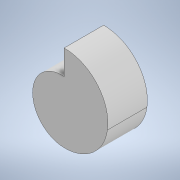
# Autodesk Inventor part: Snail Cam
Saved by Autodesk Inventor 2021 (Build 250183000, 183)
## iProperties
Created: 2021-03-30
Part Number: Snail Cam
Material: Generic
Document SubType Name: Modeling
Designer: Nabeel Azafer
Density: 1 g/cm^3
Appearance: Default
Author: Nabeel Azafer
Autodesk Inventor part; units mm, degrees
ref_plane "YZ Plane" through (0, 0, 0) normal (1, 0, 0) x (0, 1, 0)
ref_plane "XZ Plane" through (0, 0, 0) normal (0, 1, 0) x (-1, 0, 0)
ref_plane "XY Plane" through (0, 0, 0) normal (0, 0, 1) x (1, 0, 0)
sketch "Sketch2" plane through (0, 0, 0) normal (0, 0, 1) x (1, 0, 0)
  circle A0 centre (0, 0) radius 5 construction
  circle A1 centre (0, 0) radius 2.5 construction
  circle A2 centre (0, 0) radius 3.125 construction
  circle A3 centre (0, 0) radius 3.75 construction
  circle A4 centre (0, 0) radius 4.375 construction
  arc A5 (4.375, 0) -> (-0.0123, 5) centre (0.032, 0.6141) ccw
  arc A6 (0, -3.75) -> (4.375, 0) centre (0.0571, 0.6105) ccw
  arc A7 (-3.1163, 0.2327) -> (0, -3.75) centre (0.0424, -0.5062) ccw
  arc A8 (-0.0123, 2.5) -> (-3.1163, 0.2327) centre (-0.2458, -0.4388) ccw
  line L0 (-0.0123, 5) -> (-0.0123, 2.5)
  dimension "d6" = 5
  dimension "d7" = 2.5
  dimension "d9" = 0.625
  dimension "d10" = 1.25
  dimension "d11" = 1.875
  constraints: 8 point on circle, 4 centre point, 4 coincident, 3 tangent, 2 end point, 1 horizontal alignment, 1 vertical, 1 vertical alignment, 13 other
extrude "Extrusion1" add sketch "Sketch2" along normal blind 4
body "Solid1"
